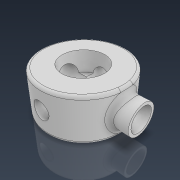
# Autodesk Inventor part: 0304_練習
Saved by Autodesk Inventor 2022 (Build 260153000, 153)
## iProperties
Created: 2022-03-04
Part Number: 0304_練習
Material: 一般
Document SubType Name: Modeling
Designer: user
Density: 1 g/cm^3
Appearance: 預設
Author: user
Autodesk Inventor part; units mm, degrees
ref_plane "XZ Plane" through (0, 0, 0) normal (0, 1, 0) x (-1, 0, 0)
sketch "草圖1" plane through (0, 0, 0) normal (0, 0, 1) x (1, 0, 0)
  line L0 (15, 15) -> (30, 15)
  line L1 (30, 15) -> (30, -15)
  line L2 (30, -15) -> (15, -15)
  line L3 (15, -15) -> (15, 15)
  line L4 (0, -21) -> (0, 21) projected
  line L5 (0, 7.5) -> (15, 7.5)
  line L6 (15, 7.5) -> (15, -7.5)
  line L7 (15, -7.5) -> (0, -7.5)
  line L8 (0, -7.5) -> (0, 7.5)
  line L9 (0, 7.5) -> (15, 7.5)
  line L10 (15, 7.5) -> (15, -15)
  line L11 (15, -15) -> (0, -15)
  line L12 (0, -15) -> (0, 7.5)
  line L13 (0, 0) -> (15, 0)
  point P0 (15, 7.5)
  point P1 (0, -15)
  dimension "d0" = 15
  dimension "d1" = 30
  dimension "d2" = 15
  dimension "d12" = 15
  dimension "d13" = 15
  constraints: 26 end point, 6 parallel, 4 perpendicular, 3 horizontal, 2 midpoint, 1 horizontal alignment
  measures "d0" distance of L1.end L2.end
  measures "d1" distance of L0.end L1.end
  measures "d2" distance of L13.start L13.end
  measures "d12" distance of L6.end L7.end
  measures "d13" distance of L5.end L6.end
revolve "迴轉1" add sketch "草圖1" angle 360 about axis through (0, -10, 0) along (0, 1, 0) contours L0 L1 L2 L3 | L3 L7 L4 L13 | L11 L4 L7 L3
ref_plane "工作平面1" through (0, 0, 30) normal (0, 0, 1) x (1, 0, 0)
sketch "草圖3" plane through (0, 0, 30) normal (0, 0, 1) x (1, 0, 0)
  circle A0 centre (0, 0) radius 6
  dimension "d11" = 12
  constraints: 1 centre point, 1 coincident
  measures "d11" diameter of A0
extrude "擠出1" cut sketch "草圖3" against normal through all
ref_plane "工作平面3" through (40, 0, 0) normal (1, 0, 0) x (0, 1, 0)
ref_plane "工作平面2" through (30, 0, 0) normal (1, 0, 0) x (0, 1, 0)
sketch "草圖4" plane through (40, 0, 0) normal (1, 0, 0) x (0, 1, 0)
  circle A0 centre (0, 0) radius 10
  circle A1 centre (0, 0) radius 8
  dimension "d18" = 20
  dimension "d19" = 2
  constraints: 2 centre point, 1 coincident
  measures "d18" diameter of A0
  measures "d19" radial gap between concentric circles of A0 A1
extrude "擠出2" add sketch "草圖4" against normal up to next
fillet "圓角1" radius 4 2 edges at (28.2843, 0.001, -10) (28.2843, -0.001, 10)
extrude "擠出3" cut sketch "草圖4" against normal through all contours A1
fillet "圓角2" radius 2 2 edges at (-30, -15, 0) (-30, 15, 0)
